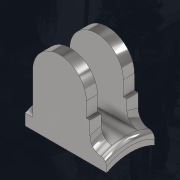
# Autodesk Inventor part: Clip
Saved by Autodesk Inventor 2021 (Build 250183000, 183)
## iProperties
Created: 2021-01-09
Part Number: Clip
Material: Generic
Document SubType Name: Modeling
Designer: Alex
Density: 1 g/cm^3
Appearance: Default
Author: Alex
Autodesk Inventor part; units mm, degrees
ref_plane "YZ Plane" through (0, 0, 0) normal (1, 0, 0) x (0, 1, 0)
ref_plane "XZ Plane" through (0, 0, 0) normal (0, 1, 0) x (-1, 0, 0)
ref_plane "XY Plane" through (0, 0, 0) normal (0, 0, 1) x (1, 0, 0)
sketch "Sketch1" plane through (0, 0, 0) normal (1, 0, 0) x (0, 1, 0)
  line L0 (1.5, 6.5) -> (-1.5, 6.5) construction
  line L1 (-1.5, 6.5) -> (-1.6004, 6.5) construction
  line L2 (1.5, -6.5) -> (-1.5, -6.5) construction
  line L3 (-1.5, -6.5) -> (-1.6004, -6.5) construction
  arc A0 (-1.6004, -6.5) -> (-1.6004, 6.5) centre (-14, 0) ccw
  arc A1 (1.5, -6.5) -> (1.5, 6.5) centre (-11.8333, 0) ccw
  arc A2 (1.5, -6.5) -> (1.5, 6.5) centre (-11.8333, 0) ccw
  line L4 (1.5, -6.5) -> (-1.6004, -6.5)
  line L5 (1.5, 6.5) -> (-1.6004, 6.5)
  point P0 (0, 0)
  point P1 (0, 0)
  constraints: 12 end point, 7 point on circle, 3 centre point, 1 collinear
extrude "Extrusion1" add sketch "Sketch1" along normal blind 22
sketch "Sketch2" plane through (0, -1.6004, 6.5) normal (0, 0, 1) x (1, 0, 0)
  line L0 (2, 3.1004) -> (0, 3.1004)
  line L1 (2, 14.1004) -> (2, 3.1004)
  line L2 (2, 3.1004) -> (2, 14.1004)
  line L3 (16.5, 10.1004) -> (16.5, 14.1004)
  line L4 (16.5, 14.1004) -> (16.5, 10.1004)
  line L5 (16.5, 10.1004) -> (17.5, 10.1004)
  line L6 (16.5, 10.1004) -> (17.5, 10.1004)
  line L7 (17.5, 3.1004) -> (22, 3.1004)
  line L8 (17.5, 10.1004) -> (17.5, 3.1004)
  arc A0 (16.5, 14.1004) -> (2, 14.1004) centre (9.25, 14.1004) ccw
  line L9 (0, 1.6004) -> (0, 0) projected
  line L10 (0, 0) -> (0, 14.7425)
  line L11 (0, 3.1004) -> (0, 4.6004) construction
  line L12 (0, 3.1004) -> (-6.4438, 3.1004) construction
  line L13 (0, 3.1004) -> (6.4438, 3.1004) construction
  line L14 (2, 3.1004) -> (17.5, 3.1004)
  dimension "d2" = 180
  constraints: 26 end point, 4 collinear, 2 perpendicular, 2 point on circle, 1 centre point, 1 horizontal, 1 tangent, 1 vertical
  measures "d2" angle of L13 L12
extrude "Extrusion2" add sketch "Sketch2" against normal up to surface (13 mm away)
sketch "Sketch3" plane through (2, 1.5, 6.5) normal (-1, 0, 0) x (0, 0, 1)
  line L0 (0, 0) -> (0, -3)
  line L1 (-13, 11) -> (-13, 18.25)
  line L2 (0, 0) -> (-13, 0)
  line L3 (-13, 0) -> (-13, 18.25)
  line L4 (-13, 18.25) -> (0, 18.25)
  line L5 (0, 18.25) -> (0, 0)
  arc A0 (0, 0) -> (-13, 0) centre (-6.5, -13.3333) ccw
  arc A1 (0, 0) -> (-13, 0) centre (-6.5, -13.3333) ccw
  line L6 (-10, 1.0812) -> (-10, 7)
  line L7 (-10, 1.0812) -> (-10, 18.25)
  line L8 (-2.9979, 11) -> (-2.9979, 18.25)
  line L9 (-2.9979, 1.0807) -> (-2.9979, 18.25)
  point P0 (-6.5, -1.5)
  point P1 (-2.9979, 1.0807)
  constraints: 20 end point, 5 point on circle, 2 centre point, 2 parallel, 2 perpendicular, 1 collinear, 1 horizontal, 1 point on line
extrude "Extrusion3" cut sketch "Sketch3" against normal blind 22 contours L4 L8 L9 A0 L6 L7
fillet "Fillet1" radius 1.5 1 edges at (22, 3, 0)
fillet "Fillet2" radius 3 2 edges at (17.5, 2.1211, 5.0302) (17.5, 2.1214, -5.0291)
sketch "Sketch4" plane through (0, 0, 0) normal (0, 1, 0) x (-1, 0, 0)
  line L0 (0, 0) -> (-7.5, 0)
  line L1 (-5.5, -2) -> (-9.5, -2)
  line L2 (-9.5, -2) -> (-9.5, 2)
  line L3 (-9.5, 2) -> (-5.5, 2)
  line L4 (-5.5, 2) -> (-5.5, -2)
  dimension "d9" = 7.5
  dimension "d10" = 4
  dimension "d11" = 4
  constraints: 10 end point, 2 horizontal, 2 parallel, 1 perpendicular
  measures "d9" distance of L0.start L0.end
  measures "d10" distance of L2.end L3.end
  measures "d11" distance of L1.end L2.end
extrude "Extrusion4" add sketch "Sketch4" along normal blind 0.5 and the other way blind 1
sketch "Sketch5" plane through (0, -1, 0) normal (0, -1, 0) x (1, 0, 0)
  line L0 (9.5, 2) -> (9.5, -2) projected
  line L1 (5.5, -2) -> (5.5, 2) projected
  line L2 (9.5, -2) -> (5.5, -2)
  line L3 (5.5, -2) -> (5.5, 2)
  line L4 (5.5, 2) -> (9.5, 2)
  line L5 (9.5, 2) -> (9.5, -2)
  point P0 (0, 0)
  constraints: 8 end point, 2 parallel, 1 horizontal, 1 perpendicular
extrude "Extrusion5" add sketch "Sketch5" along normal up to surface (0.6004 mm away)
sketch "Sketch6" plane through (5.5, -1.6004, -2) normal (0, -1, 0) x (1, 0, 0)
  line L0 (0, 4) -> (4, 4) projected
  line L1 (0, 0) -> (4, 0)
  line L2 (4, 0) -> (4, 4)
  line L3 (4, 4) -> (0, 4)
  line L4 (0, 4) -> (0, 0)
  point P0 (-5.5, 2)
  constraints: 8 end point, 2 parallel, 1 horizontal, 1 perpendicular
extrude "Extrusion6" cut sketch "Sketch6" against normal blind 0.6
body "Solid1"
